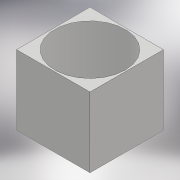
# Autodesk Inventor part: TestTubeSocket
Saved by Autodesk Inventor 2018 (Build 220112000, 112)
## iProperties
Created: 2019-05-03
Part Number: TestTubeSocket
Material: Generic
Document SubType Name: Modeling
Designer: Isaac Newcomb
Density: 1 g/cm^3
Appearance: Default
Author: Isaac Newcomb
Autodesk Inventor part; units mm, degrees
ref_plane "YZ Plane" through (0, 0, 0) normal (1, 0, 0) x (0, 1, 0)
ref_plane "XZ Plane" through (0, 0, 0) normal (0, 1, 0) x (-1, 0, 0)
ref_plane "XY Plane" through (0, 0, 0) normal (0, 0, 1) x (1, 0, 0)
sketch "Sketch1" plane through (0, 0, 0) normal (0, 0, 1) x (1, 0, 0)
  circle A0 centre (0, 0) radius 5.05
  line L0 (-5.25, -5.25) -> (5.25, -5.25)
  line L1 (5.25, -5.25) -> (5.25, 5.25)
  line L2 (5.25, 5.25) -> (-5.25, 5.25)
  line L3 (-5.25, 5.25) -> (-5.25, -5.25)
  line L4 (-5.25, -5.25) -> (5.25, 5.25) construction
  line L5 (5.25, -5.25) -> (-5.25, 5.25) construction
  dimension "d0" = 10.1
  dimension "d1" = 10.5
  dimension "d2" = 10.5
  constraints: 12 end point, 2 midpoint, 2 parallel, 1 centre point, 1 coincident, 1 horizontal, 1 perpendicular
  measures "d0" diameter of A0
  measures "d1" distance of L2.end L1.end
  measures "d2" distance of L1.end L0.end
extrude "Extrusion1" add sketch "Sketch1" along normal blind 10
body "Solid1"
